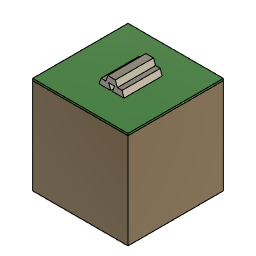
Tree gone with Ore v1 (Autodesk Fusion 360 design; units mm, degrees)
Autodesk Fusion 360 part; units mm, degrees
sketch "Skizze1" plane through (0, 0, 0) normal (0, 0, 1) x (1, 0, 0)
  line L0 (0, 0) -> (50, 0)
  line L1 (50, 0) -> (50, 50)
  line L2 (50, 50) -> (0, 50)
  line L3 (0, 50) -> (0, 0)
  line L4 (20, 20) -> (5, 20)
  line L5 (5, 20) -> (5, 5)
  line L6 (5, 5) -> (20, 5)
  line L7 (20, 5) -> (20, 20)
  line L8 (20, 40) -> (35, 40)
  line L9 (35, 40) -> (35, 25)
  line L10 (35, 25) -> (30, 25)
  line L11 (30, 25) -> (30, 30)
  line L12 (30, 30) -> (20, 30)
  line L13 (20, 30) -> (20, 40)
  line L14 (5, 45) -> (15, 45)
  line L15 (15, 45) -> (15, 35)
  line L16 (15, 35) -> (5, 35)
  line L17 (5, 35) -> (5, 45)
  line L18 (30, 15) -> (40, 15)
  line L19 (40, 15) -> (40, 5)
  line L20 (40, 5) -> (30, 5)
  line L21 (30, 5) -> (30, 15)
  line L22 (40, 40) -> (45, 40)
  line L23 (45, 40) -> (45, 30)
  line L24 (45, 30) -> (40, 30)
  line L25 (40, 30) -> (40, 40)
  constraint coincident L0.start L3.end
  constraint horizontal L4
  constraint vertical L5
  constraint horizontal L6
  constraint vertical L7
  constraint horizontal L8
  constraint perpendicular L8 L9
  constraint perpendicular L9 L10
  constraint perpendicular L10 L11
  constraint perpendicular L11 L12
  constraint perpendicular L12 L13
  constraint coincident L8.start L13.end
  constraint horizontal L14
  constraint vertical L15
  constraint horizontal L16
  constraint vertical L17
  constraint horizontal L18
  constraint vertical L19
  constraint horizontal L20
  constraint vertical L21
  constraint horizontal L22
  constraint vertical L23
  constraint horizontal L24
  constraint vertical L25
extrude "Extrusion1" add sketch "Skizze1" along normal blind 25 contours L4 L5 L6 L7 makes body 1 in component "Großer Block"
extrude "Extrusion1'" add sketch "Skizze1" along normal blind 15 separate body contours L18 L19 L20 L21 makes body 2 in component "Medium Block 1"
extrude "Extrusion1''" add sketch "Skizze1" along normal blind 15 separate body contours L14 L15 L16 L17 makes body 3 in component "Medium Block 2#"
extrude "Extrusion1'''" add sketch "Skizze1" along normal blind 10 separate body contours L8 L9 L10 L11 L12 L13 makes body 4 in component "L Block"
extrude "Extrusion1''''" add sketch "Skizze1" along normal blind 5 separate body contours L22 L23 L24 L25 makes body 5 in component "Smal Block 1"
extrude "Extrusion1'''''" add sketch "Skizze1" against normal blind 1 separate body contours L0 L1 L2 L3 | L4 L5 L6 L7 | L8 L9 L10 L11 L12 L13 | L14 L15 L16 L17 | L18 L19 L20 L21 | L22 L23 L24 L25 makes body 6 in component "Boden"
extrude "Extrusion1''''''" add 1 faces at (16.6667, 33.3333, -1) along direction (0, 0, -1) blind 50 separate body on bodies 6 makes body 7 in component "Ground below"
ref_plane "Arbeitsebene1" through (25, 25, -26) normal (0, -1, 0) x (-1, 0, 0)
sketch "Skizze4" plane through (25, 25, -26) normal (0, -1, 0) x (1, 0, 0)
  line L0 (-5.1085, 26) -> (-4.1085, 29)
  line L1 (-4.1085, 29) -> (-0.1085, 29)
  line L2 (-0.1085, 29) -> (0.8915, 26)
  line L3 (0.8915, 26) -> (-5.1085, 26)
  line L4 (6.8915, 29) -> (7.8915, 26)
  line L5 (1.8915, 26) -> (2.8915, 29)
  line L6 (2.8915, 29) -> (6.8915, 29)
  line L7 (7.8915, 26) -> (1.8915, 26)
  line L8 (3.3915, 32) -> (4.3915, 29)
  line L9 (-1.6085, 29) -> (-0.6085, 32)
  line L10 (-0.6085, 32) -> (3.3915, 32)
  line L11 (4.3915, 29) -> (-1.6085, 29)
  line L12 (-25, 26) -> (25, 26)
  dimension "d20" = 4
  dimension "d21" = 6
  dimension "d22" = 1
  dimension "d23" = 3
  dimension "d32" = 6
  dimension "d33" = 4
  dimension "d34" = 1
  dimension "d35" = 3
  dimension "d36" = 6
  dimension "d37" = 4
  dimension "d38" = 1
  dimension "d39" = 3
  dimension "d40" = 1
  dimension "d41" = 1.5
  constraint horizontal L1
  constraint parallel L1 L3
  constraint horizontal L6
  constraint parallel L6 L7
  constraint horizontal L10
  constraint parallel L10 L11
  constraint collinear L7 L12
  constraint collinear L3 L12
  constraint collinear L6 L11
  measures "d20" distance of L0.end L1.end
  measures "d21" distance of L0.start L2.end
  measures "d22" horizontal distance of L0.start L0.end
  measures "d23" distance of L0.end L3
  measures "d32" distance of L4.end L5.start
  measures "d33" distance of L5.end L4.start
  measures "d34" horizontal distance of L5.start L5.end
  measures "d35" vertical distance of L5.start L5.end
  measures "d36" distance of L8.end L9.start
  measures "d37" distance of L9.end L8.start
  measures "d38" horizontal distance of L9.start L9.end
  measures "d39" vertical distance of L9.start L9.end
  measures "d40" distance of L2.end L5.start
  measures "d41" distance of L1.end L9.start
extrude "Extrusion1'''''''" add sketch "Skizze4" along normal mid plane 20 separate body contours L0 L1 L2 L3 L11 L12 | L1 L6 L8 L9 L10 L11 | L4 L5 L6 L7 L11 L12 makes body 8 in component "Ore"
component "Großer Block" placed x (1, 0, 0) y (0, 1, 0) z (0, 0, 1) at (0, 0, 0)
component "Medium Block 1" placed x (1, 0, 0) y (0, 1, 0) z (0, 0, 1) at (0, 0, 0)
component "Medium Block 2#" placed x (1, 0, 0) y (0, 1, 0) z (0, 0, 1) at (0, 0, 0)
component "L Block" placed x (1, 0, 0) y (0, 1, 0) z (0, 0, 1) at (0, 0, 0)
component "Smal Block 1" placed x (1, 0, 0) y (0, 1, 0) z (0, 0, 1) at (0, 0, 0)
component "Boden" placed x (1, 0, 0) y (0, 1, 0) z (0, 0, 1) at (0, 0, 0)
component "Ground below" placed x (1, 0, 0) y (0, 1, 0) z (0, 0, 1) at (0, 0, 0)
component "Ore" placed x (1, 0, 0) y (0, 1, 0) z (0, 0, 1) at (0, 0, 0)
equation "d32 = d21"
equation "d33 = d20"
equation "d34 = d22"
equation "d35 = d23"
equation "d36 = d21"
equation "d37 = d20"
equation "d38 = d22"
equation "d39 = d23"
equation "d41 = ( d36 - d40 ) / 2 - d22"
